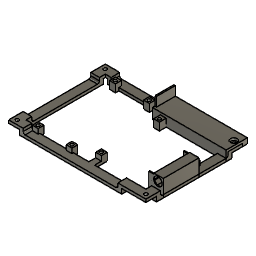
sensor_mounting (Autodesk Fusion 360 design; units mm, degrees)
Autodesk Fusion 360 part; units mm, degrees
note: some values were not read from the file. Set by a fixed rule: which sketch regions a step uses.
sketch "Skizze1" plane through (0, 0, 0) normal (0, 0, 1) x (1, 0, 0)
  line L0 (0, 0) -> (142, 0)
  line L1 (142, 0) -> (142, 100)
  line L2 (142, 100) -> (0, 100)
  line L3 (0, 100) -> (0, 0)
  line L4 (133, 9) -> (133, 91)
  line L5 (133, 91) -> (9, 91)
  line L6 (9, 91) -> (9, 9)
  line L7 (9, 9) -> (133, 9)
  circle A0 centre (4.5, 95.5) radius 1.75
  circle A1 centre (137.5, 95.5) radius 1.75
  circle A2 centre (137.5, 4.5) radius 1.75
  circle A3 centre (4.5, 4.5) radius 1.75
  line L8 (11, 91) -> (11, 100)
  line L9 (11, 0) -> (11, 1)
  line L10 (11, 1) -> (11, 9)
  line L11 (117, 9) -> (117, 0)
  line L12 (15, 91) -> (15, 100)
  line L13 (113, 100) -> (113, 91)
  line L14 (113, 9) -> (113, 0)
  line L15 (15, 0) -> (15, 9)
  line L16 (117, 91) -> (117, 100)
  line L17 (0, 11) -> (9, 11)
  line L18 (0, 15) -> (9, 15)
  line L19 (0, 89) -> (9, 89)
  line L20 (9, 85) -> (0, 85)
  line L21 (133, 89) -> (142, 89)
  line L22 (142, 85) -> (133, 85)
  line L23 (133, 11) -> (142, 11)
  line L24 (133, 15) -> (142, 15)
  line L25 (9, 41) -> (9, 50)
  circle A4 centre (132, 60) radius 1.6
  circle A5 centre (77, 79) radius 1.6
  circle A6 centre (77, 19) radius 1.6
  line L26 (129, 63) -> (133, 63)
  line L27 (133, 63) -> (133, 57)
  line L28 (133, 57) -> (129, 57)
  line L29 (129, 57) -> (129, 63)
  line L30 (74, 22) -> (80, 22)
  line L31 (80, 22) -> (80, 9)
  line L32 (80, 9) -> (74, 9)
  line L33 (74, 9) -> (74, 22)
  line L34 (80, 91) -> (74, 91)
  line L35 (74, 91) -> (74, 76)
  line L36 (74, 76) -> (80, 76)
  line L37 (80, 76) -> (80, 91)
  line L38 (135, 63) -> (135, 57)
  line L39 (74, 82) -> (80, 82)
  line L40 (74, 16) -> (80, 16)
  circle A7 centre (55, 90.5499) radius 1.6
  line L41 (55, 90.5499) -> (55, 44) construction
  circle A8 centre (55, 10.5499) radius 1.6
  line L42 (55, 10.5499) -> (28.4536, 10.5499) construction
  circle A9 centre (20, 10.5499) radius 1.6
  line L43 (20, 10.5499) -> (20, 84) construction
  circle A10 centre (20, 90.5499) radius 1.6
  line L44 (58, 87.5499) -> (52, 87.5499)
  line L45 (52, 87.5499) -> (52, 93.5499)
  line L46 (52, 93.5499) -> (58, 93.5499)
  line L47 (58, 93.5499) -> (58, 87.5499)
  line L48 (58, 87.5499) -> (52, 93.5499) construction
  line L49 (52, 87.5499) -> (58, 93.5499) construction
  line L50 (23, 87.5499) -> (17, 87.5499)
  line L51 (17, 87.5499) -> (17, 93.5499)
  line L52 (17, 93.5499) -> (23, 93.5499)
  line L53 (23, 93.5499) -> (23, 87.5499)
  line L54 (23, 87.5499) -> (17, 93.5499) construction
  line L55 (17, 87.5499) -> (23, 93.5499) construction
  line L56 (58, 7.5499) -> (52, 7.5499)
  line L57 (52, 7.5499) -> (52, 13.5499)
  line L58 (52, 13.5499) -> (58, 13.5499)
  line L59 (58, 13.5499) -> (58, 7.5499)
  line L60 (58, 7.5499) -> (52, 13.5499) construction
  line L61 (52, 7.5499) -> (58, 13.5499) construction
  line L62 (23, 7.5499) -> (17, 7.5499)
  line L63 (17, 7.5499) -> (17, 13.5499)
  line L64 (17, 13.5499) -> (23, 13.5499)
  line L65 (23, 13.5499) -> (23, 7.5499)
  line L66 (23, 7.5499) -> (17, 13.5499) construction
  line L67 (17, 7.5499) -> (23, 13.5499) construction
  line L68 (77, 79) -> (155, 79) construction
  line L69 (142, 19) -> (130.2, 19)
  line L70 (130.2, 19) -> (130.2, 54)
  line L71 (130.2, 54) -> (142, 54)
  line L72 (142, 54) -> (142, 19)
  line L73 (142, 54) -> (127, 54)
  line L74 (127, 54) -> (127, 55)
  line L75 (127, 55) -> (142, 55)
  line L76 (142, 55) -> (142, 54)
  line L77 (142, 19) -> (127, 19)
  line L78 (127, 19) -> (127, 18)
  line L79 (127, 18) -> (142, 18)
  line L80 (142, 18) -> (142, 19)
  line L81 (129.2, 54) -> (129.2, 19)
  line L82 (133, 57) -> (135, 57)
  line L83 (133, 63) -> (135, 63)
  line L84 (142, 54) -> (141, 54)
  line L85 (141, 54) -> (141, 19)
  line L86 (141, 19) -> (142, 19)
  line L87 (142, 19) -> (142, 54)
  line L88 (142, 83) -> (66, 83)
  line L89 (66, 83) -> (66, 105)
  line L90 (66, 105) -> (142, 105)
  line L91 (142, 105) -> (142, 83)
  line L92 (67.5, 83) -> (67.5, 105)
  line L93 (113, 100) -> (113, 105)
  line L94 (117, 100) -> (117, 105)
  line L95 (133, 89) -> (117, 89)
  line L96 (117, 91) -> (117, 89)
  line L97 (66, 85.5) -> (67.5, 85.5)
  point P0 (55, 90.5499)
  point P1 (20, 90.5499)
  point P2 (55, 10.5499)
  point P3 (20, 10.5499)
  dimension "d1" = 142
  dimension "d2" = 100
  dimension "d3" = -9
  dimension "d4" = 4.5
  dimension "d5" = 4.5
  dimension "d6" = 3.5
  dimension "d7" = 3.5
  dimension "d8" = 3.5
  dimension "d9" = 3.5
  dimension "d10" = 4.5
  dimension "d11" = 4.5
  dimension "d12" = 4.5
  dimension "d13" = 4.5
  dimension "d14" = 4.5
  dimension "d15" = 4.5
  dimension "d17" = 11
  dimension "d18" = 11
  dimension "d19" = 25
  dimension "d20" = 4
  dimension "d21" = 4
  dimension "d23" = 4
  dimension "d24" = 25
  dimension "d25" = 4
  dimension "d43" = 11
  dimension "d44" = 4
  dimension "d45" = 11
  dimension "d46" = 4
  dimension "d47" = 11
  dimension "d48" = 4
  dimension "d49" = 11
  dimension "d50" = 4
  dimension "d63" = 3.2
  dimension "d64" = 3.2
  dimension "d66" = 55
  dimension "d67" = 3.2
  dimension "d69" = 60
  dimension "d70" = 55
  dimension "d85" = 3
  dimension "d86" = 3
  dimension "d87" = 3
  dimension "d88" = 3
  dimension "d89" = 3
  dimension "d90" = 3
  dimension "d91" = 3
  dimension "d92" = 3
  dimension "d93" = 3
  dimension "d94" = 3
  dimension "d95" = 3
  dimension "d96" = 3
  dimension "d100" = 3.2
  dimension "d102" = 3.2
  dimension "d103" = 3.2
  dimension "d104" = 3.2
  dimension "d105" = 80
  dimension "d106" = 80
  dimension "d107" = 35
  dimension "d108" = 20
  dimension "d109" = 6
  dimension "d110" = 6
  dimension "d111" = 6
  dimension "d112" = 6
  dimension "d113" = 6
  dimension "d114" = 6
  dimension "d115" = 6
  dimension "d116" = 6
  dimension "d119" = 10
  dimension "d120" = 41
  dimension "d128" = 10
  dimension "d131" = 19
  dimension "d132" = 35
  dimension "d133" = 11.8
  dimension "d134" = 1
  dimension "d135" = 15
  dimension "d136" = 1
  dimension "d137" = 15
  dimension "d138" = 1
  dimension "d143" = 1
  dimension "d152" = 22
  dimension "d153" = 76
  dimension "d154" = 5
  dimension "d155" = 1.5
  dimension "d166" = 2.5
  constraint horizontal L0
  constraint vertical L1
  constraint horizontal L2
  constraint vertical L3
  constraint coincident L0.start L3.end
  constraint coincident L5 L8.start
  constraint coincident L2 L8.end
  constraint perpendicular L2 L8
  constraint coincident L0 L9.start
  constraint perpendicular L0 L9
  constraint coincident L7 L10.end
  constraint perpendicular L7 L10
  constraint coincident L7 L11.start
  constraint coincident L0 L11.end
  constraint perpendicular L7 L11
  constraint coincident L5 L12.start
  constraint coincident L2 L12.end
  constraint perpendicular L2 L12
  constraint coincident L2 L13.start
  constraint coincident L5 L13.end
  constraint perpendicular L5 L13
  constraint coincident L7 L14.start
  constraint coincident L0 L14.end
  constraint perpendicular L0 L14
  constraint coincident L0 L15.start
  constraint coincident L7 L15.end
  constraint perpendicular L7 L15
  constraint coincident L5 L16.start
  constraint coincident L2 L16.end
  constraint perpendicular L2 L16
  constraint coincident L3 L17.start
  constraint coincident L6 L17.end
  constraint perpendicular L6 L17
  constraint coincident L3 L18.start
  constraint coincident L6 L18.end
  constraint perpendicular L6 L18
  constraint coincident L3 L19.start
  constraint coincident L6 L19.end
  constraint perpendicular L6 L19
  constraint coincident L6 L20.start
  constraint coincident L3 L20.end
  constraint perpendicular L3 L20
  constraint coincident L4 L21.start
  constraint coincident L1 L21.end
  constraint perpendicular L1 L21
  constraint coincident L1 L22.start
  constraint coincident L4 L22.end
  constraint perpendicular L4 L22
  constraint coincident L4 L23.start
  constraint coincident L1 L23.end
  constraint perpendicular L1 L23
  constraint coincident L4 L24.start
  constraint coincident L1 L24.end
  constraint perpendicular L1 L24
  constraint vertical L25
  constraint coincident L6 L25.end
  constraint horizontal L26
  constraint vertical L27
  constraint horizontal L28
  constraint vertical L29
  constraint coincident L4 L27.end
  constraint horizontal L30
  constraint vertical L31
  constraint horizontal L32
  constraint vertical L33
  constraint coincident L7 L31.end
  constraint horizontal L34
  constraint vertical L35
  constraint horizontal L36
  constraint vertical L37
  constraint coincident L5 L34.start
  constraint coincident L26 L38.start
  constraint coincident L28 L38.end
  constraint perpendicular L28 L38
  constraint coincident L35 L39.start
  constraint coincident L37 L39.end
  constraint perpendicular L37 L39
  constraint coincident L33 L40.start
  constraint coincident L31 L40.end
  constraint perpendicular L31 L40
  constraint coincident P0 A7.centre
  constraint vertical L41
  constraint coincident L41 P2
  constraint coincident P2 A8.centre
  constraint perpendicular L41 L42
  constraint coincident L42 P3
  constraint coincident P3 A9.centre
  constraint perpendicular L42 L43
  constraint coincident L43 P1
  constraint horizontal L44
  constraint perpendicular L44 L45
  constraint parallel L44 L46
  constraint parallel L45 L47
  constraint coincident L48 P0
  constraint coincident L49 P0
  constraint horizontal L50
  constraint perpendicular L50 L51
  constraint parallel L50 L52
  constraint parallel L51 L53
  constraint coincident L54 P1
  constraint coincident L55 P1
  constraint coincident P1 A10.centre
  constraint horizontal L56
  constraint perpendicular L56 L57
  constraint parallel L56 L58
  constraint parallel L57 L59
  constraint coincident L60 P2
  constraint coincident L61 P2
  constraint horizontal L62
  constraint perpendicular L62 L63
  constraint parallel L62 L64
  constraint parallel L63 L65
  constraint coincident L66 P3
  constraint coincident L67 P3
  constraint coincident A5.centre L68.start
  constraint perpendicular L1 L68
  constraint horizontal L69
  constraint vertical L70
  constraint horizontal L71
  constraint vertical L72
  constraint coincident L1 L69.start
  constraint horizontal L73
  constraint vertical L74
  constraint horizontal L75
  constraint vertical L76
  constraint horizontal L77
  constraint vertical L78
  constraint horizontal L79
  constraint vertical L80
  constraint coincident L73 L81.start
  constraint coincident L77 L81.end
  constraint perpendicular L77 L81
  constraint horizontal L84
  constraint vertical L85
  constraint horizontal L86
  constraint vertical L87
  constraint coincident L77 L85.end
  constraint horizontal L88
  constraint vertical L89
  constraint horizontal L90
  constraint vertical L91
  constraint coincident L1 L88.start
  constraint coincident L88 L92.start
  constraint coincident L90 L92.end
  constraint perpendicular L90 L92
  constraint coincident L90 L93.end
  constraint perpendicular L90 L93
  constraint coincident L90 L94.end
  constraint perpendicular L90 L94
  constraint perpendicular L4 L95
  constraint perpendicular L95 L96
  constraint coincident L89 L97.start
  constraint coincident L92 L97.end
  constraint perpendicular L92 L97
  measures "d1" distance of L1.end L2.end
  measures "d2" distance of L0.start L2.end
  measures "d4" distance of L3 A0.centre
  measures "d5" distance of L2 A0.centre
  measures "d6" diameter of A0
  measures "d7" diameter of A3
  measures "d8" diameter of A2
  measures "d9" diameter of A1
  measures "d10" distance of L1 A1.centre
  measures "d11" distance of L2 A1.centre
  measures "d12" distance of L1 A2.centre
  measures "d13" distance of L0 A2.centre
  measures "d14" distance of L3 A3.centre
  measures "d15" distance of L0 A3.centre
  measures "d17" distance of L2.end L8.end
  measures "d18" distance of L0.start L9.start
  measures "d19" distance of L0.end L11.end
  measures "d20" distance of L10.end L15.end
  measures "d21" distance of L11.start L14.start
  measures "d23" distance of L8.start L12.start
  measures "d24" distance of L1 L16
  measures "d25" distance of L13.start L16.end
  measures "d43" distance of L0.start L17.start
  measures "d44" distance of L17.start L18.start
  measures "d45" distance of L2.end L19.start
  measures "d46" distance of L19.start L20.end
  measures "d47" distance of L1.end L21.end
  measures "d48" distance of L21.end L22.start
  measures "d49" distance of L0.end L23.end
  measures "d50" distance of L23.end L24.end
  measures "d63" diameter of A4
  measures "d64" diameter of A5
  measures "d66" horizontal distance of A4.centre A5.centre
  measures "d67" diameter of A6
  measures "d69" vertical distance of A5.centre A6.centre
  measures "d70" horizontal distance of A4.centre A6.centre
  measures "d85" distance of A4.centre L26
  measures "d86" distance of A4.centre L28
  measures "d87" distance of A4.centre L29
  measures "d88" distance of A6.centre L30
  measures "d89" distance of A6.centre L31
  measures "d90" distance of A6.centre L33
  measures "d91" distance of A5.centre L37
  measures "d92" distance of A5.centre L35
  measures "d93" distance of A5.centre L36
  measures "d94" distance of A4.centre L38
  measures "d95" distance of A5.centre L39
  measures "d96" distance of A6.centre L40
  measures "d103" diameter of A9
  measures "d104" diameter of A10
  measures "d105" distance of P0 P2
  measures "d106" distance of P3 P1
  measures "d107" distance of P2 P3
  measures "d108" distance of L3 P1
  measures "d109" distance of L45.end L46.end
  measures "d110" distance of L44.end L45.end
  measures "d111" distance of L51.end L52.end
  measures "d112" distance of L50.end L51.end
  measures "d113" distance of L57.end L58.end
  measures "d114" distance of L56.end L57.end
  measures "d115" distance of L63.end L64.end
  measures "d116" distance of L62.end L63.end
  measures "d119" distance of L7 A6.centre
  measures "d120" vertical distance of A4.centre A6.centre
  measures "d128" distance of L1 A4.centre
  measures "d131" distance of L0 L69
  measures "d132" distance of L69 L71
  measures "d133" distance of L70.end L72
  measures "d134" distance of L73 L75
  measures "d135" distance of L71.end L73.end
  measures "d136" distance of L77.end L78.end
  measures "d137" distance of L78.end L79.end
  measures "d138" distance of L70 L81
  measures "d143" distance of L85 L87
  measures "d152" distance of L88.end L89.end
  measures "d153" distance of L89.end L90.end
  measures "d154" distance of L2 L90
  measures "d155" distance of L89 L92
  measures "d166" distance of L88 L97
extrude "Extrusion17" add sketch "Skizze1" along normal blind 20 contours L2 L89 L90 L92 | L2 L5 L89 L92 | L5 L89 L92 L97 makes body 1
extrude "Extrusion16" add sketch "Skizze1" along normal blind 10.5 separate body contours L2 L90 L92 L93 | L2 L5 L13 L34 L92 | L2 L90 L93 L94 | L2 L5 L13 L16 | L5 L35 L88 L92 | L88 L89 L92 L97 | L2 L90 L91 L94 | L1 L2 L4 L5 L16 L21 L91 | L4 L5 L37 L88 L95 L96 | L5 L34 L35 L37 L88 | L1 L4 L22 L88 L91 | L4 L5 L95 L96 | L1 L4 L21 L22 L91 makes body 2
extrude "Extrusion13" add sketch "Skizze1" along normal blind 16.5 separate body contours L1 L4 L69 L77 L79 L80 L86 | L1 L69 L71 L72 L73 L77 L84 L85 L86 L87 | L4 L69 L77 L78 L79 | L1 L4 L71 L73 L75 L76 L84 | L4 L71 L73 L74 L75 makes body 3
extrude "Extrusion12" add sketch "Skizze1" along normal blind 8.8 separate body contours L70 L73 L77 L81 makes body 4
extrude "Extrusion11" add sketch "Skizze1" along normal blind 8 separate body contours L7 A9 L63 L64 L65 | L7 A9 L62 L63 L65 | L7 A8 L56 L57 L59 | L7 A8 L57 L58 L59 | L5 A10 L51 L52 L53 | L5 A10 L50 L51 L53 | L5 A7 L44 L45 L47 | L5 A7 L45 L46 L47 makes body 5 at (56.598, 10.4701, 5.3333) makes body 6 at (18.9413, 89.3502, 5.3333) makes body 7 at (21.592, 10.7092, 2.6667) makes body 8 at (56.1172, 91.6953, 5.3333)
extrude "Extrusion10" add sketch "Skizze1" along normal blind 8 separate body contours L30 L31 L33 L40 | L35 L37 L39 L88 | L4 A4 L26 L27 L28 L29 | L4 A4 L27 L38 L82 L83 | L35 L36 L37 L39 makes body 9 at (77.0399, 20.5995, 5.3333) makes body 10 at (77.0399, 80.5995, 5.3333) makes body 11 at (132.1989, 58.4124, 2.6667)
extrude "Extrusion2" add sketch "Skizze1" along normal blind 8 separate body contours L0 L3 L6 L7 L9 L10 L17 | L0 L7 L9 L10 L15 | L3 L6 L17 L18 | L0 L7 L11 L14 | L3 L6 L19 L20 | L0 L1 L4 L7 L11 L23 | L2 L3 L5 L6 L8 L19 | L1 L4 L23 L24 | L2 L5 L8 L12 | L2 L5 L13 L16 | L1 L2 L4 L5 L16 L21 L91 | L1 L4 L21 L22 L91 makes body 12 at (13, 6, 0) makes body 13 at (119.6667, 6, 0) makes body 14 at (119.6667, 94, 0) makes body 15 at (6, 87, 0)
extrude "Extrusion3" add sketch "Skizze1" along normal blind 3 contours L0 L7 L14 L15 L32 L56 L57 L59 L62 L63 L65 | L3 L6 L18 L20 L25 | L7 L31 L32 L33 L40 | L7 A9 | L1 L4 L24 L79 | L2 L5 L12 L45 L46 L47 L51 L52 L53 L89 | L1 L4 L69 L77 L79 L80 L86 | L7 A8 | L2 L5 L89 L92 | L1 L69 L71 L72 L73 L77 L84 L85 L86 L87 | L2 L5 L13 L34 L92 | L1 L4 L71 L73 L75 L76 L84 | L4 L69 L71 L73 L77 L85 | L4 L69 L70 L71 L73 L77 | L1 L4 L38 L75 L82 L83 L88 | L5 L34 L35 L37 L88 | L1 L4 L22 L88 L91 | L35 L37 L39 L88 | L4 A4 L26 L27 L28 L29 | L4 A4 L27 L38 L82 L83 picked at (20.0668, 8.9875) picked at (54.9332, 8.9875) bodies 11 5 6 7 8 9 10 13 14 15 12
extrude "Extrusion4" cut sketch "Skizze1" along normal blind 5 contours L0 L3 L6 L7 L9 L10 L17 | L0 L1 L4 L7 L11 L23 | L2 L3 L5 L6 L8 L19 bodies 11
extrude "Extrusion18" cut sketch "Skizze1" along normal up to surface (5 mm away) contours L2 L90 L91 L94 | L1 L2 L4 L5 L16 L21 L91 | L4 L5 L95 L96 bodies 2 11
fillet "Abrundung2" radius 2 8 edges at (113, 4.5, 3) (113, 95.5, 3) (15, 95.5, 3) (4.5, 85, 3) (15, 4.5, 3) (4.5, 15, 3) (137.5, 15, 3) (137.5, 85, 3) on bodies 11
sketch "Skizze3" plane through (0, 18, 0) normal (0, -1, 0) x (1, 0, 0)
  line L0 (127, 0) -> (142, 0)
  line L1 (142, 0) -> (142, 16.5)
  line L2 (142, 16.5) -> (127, 16.5)
  line L3 (127, 16.5) -> (127, 0)
  circle A0 centre (136.4271, 12.0478) radius 4.4
  dimension "d146" = 8.8
  measures "d146" diameter of A0
extrude "Extrusion14" cut sketch "Skizze3" against normal up to surface (1 mm away) contours A0 bodies 3
sketch "Skizze4" plane through (0, 0, 16.5) normal (0, 0, 1) x (-1, 0, 0)
  line L0 (-141, -54) -> (-141, -19)
  line L1 (-141, -19) -> (-127, -19)
  line L2 (-127, -19) -> (-127, -18)
  line L3 (-127, -18) -> (-142, -18)
  line L4 (-142, -18) -> (-142, -55)
  line L5 (-142, -55) -> (-127, -55)
  line L6 (-127, -55) -> (-127, -54)
  line L7 (-127, -54) -> (-141, -54)
  line L8 (-132.3, -55) -> (-142, -55)
  line L9 (-142, -55) -> (-142, -18)
  line L10 (-142, -18) -> (-132.3, -18)
  line L11 (-132.3, -18) -> (-132.3, -55)
  dimension "d149" = 9.7
  constraint horizontal L8
  constraint vertical L9
  constraint horizontal L10
  constraint vertical L11
  constraint coincident L3.end L4.start
  constraint coincident L5 L8.start
  measures "d149" distance of L9 L11
extrude "Extrusion15" add sketch "Skizze4" along normal blind 1 contours L0 L1 L3 L4 L5 L7 L8 L9 L10 L11 | L0 L1 L7 L11 bodies 3
sketch "Skizze5" plane through (0, 0, 10.5) normal (0, 0, 1) x (-1, 0, 0)
  circle A0 centre (-137.5, -95.5) radius 1.75
  line L0 (-66, -83) -> (-142, -83)
  line L1 (-142, -83) -> (-142, -105)
  line L2 (-142, -105) -> (-67.5, -105)
  line L3 (-67.5, -105) -> (-67.5, -85.5)
  circle A1 centre (-137.5, -95.5) radius 3.5
  line L4 (-66, -85.5) -> (-66, -83)
  line L5 (-67.5, -85.5) -> (-66, -85.5)
  dimension "d163" = 7
  constraint concentric A0 A1
  measures "d163" diameter of A1
extrude "Extrusion19" cut sketch "Skizze5" against normal up to surface (2.5 mm away) contours A1 bodies 2
equation "d63 = bohrung_abstanzbolzen"
equation "d64 = bohrung_abstanzbolzen"
equation "d67 = bohrung_abstanzbolzen"
equation "d100 = bohrung_abstanzbolzen"
equation "d102 = bohrung_abstanzbolzen"
equation "d103 = bohrung_abstanzbolzen"
equation "d104 = bohrung_abstanzbolzen"
equation "bohrung_abstanzbolzen = 3.2 mm"
equation "d133 = 15.8 mm - 4 mm"
equation "d141 = 7.7 mm + 8.8 mm"
equation "d149 = 11.8 mm - 2.1 mm"
